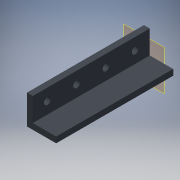
# Autodesk Inventor part: inside Angle beam
Saved by Autodesk Inventor 2016 (Build 200138000, 138)
## iProperties
Created: 2015-08-29
Part Number: inside Angle beam
Material: Generic
Description: ANGLE - 144 MM
Document SubType Name: Modeling
Designer: PTC
Density: 1 g/cm^3
Appearance: Default
Sending System: Creo  TM  2.0  (c) 2012
PROJECT: FTC
PTC_MATERIAL_NAME: METAL_ALUMINIUM_5052
NIKCONFIGCOUNT: 1
KIT: TETRIX
Author: phi
Autodesk Inventor part; units mm, degrees
ref_plane "FRONT" through (0, 0, 0) normal (0, 0, 1) x (1, 0, 0)
ref_plane "TOP" through (0, 0, 0) normal (0, 1, 0) x (-1, 0, 0)
ref_plane "RIGHT" through (0, 0, 0) normal (1, 0, 0) x (0, 1, 0)
ref_plane "Work Plane4" through (0, 0, 0) normal (0, 0, 1) x (1, 0, 0)
sketch "Sketch1" plane through (0, 0, 0) normal (0, 0, 1) x (1, 0, 0)
  line L0 (3.2, 16) -> (0, 16) projected
  line L1 (3.2, 3.2) -> (3.2, 14) projected
  line L2 (3.2, 14) -> (3.2, 16) projected
  line L3 (0, 16) -> (0, 14) projected
  line L4 (0, 14) -> (0, 0) projected
  line L5 (0, 0) -> (14, 0) projected
  line L6 (16, 0) -> (16, 3.2) projected
  line L7 (16, 3.2) -> (14, 3.2) projected
  line L8 (14, 3.2) -> (3.2, 3.2) projected
  line L9 (14, 0) -> (16, 0) projected
extrude "Extrusion1" add sketch "Sketch1" along normal blind 80
sketch "Sketch2" plane through (0, 0, 0) normal (-1, 0, 0) x (0, 0, 1)
  circle A0 centre (8, 9.6) radius 1.85 projected
  circle A1 centre (24, 9.6) radius 1.85 projected
  circle A2 centre (40, 9.6) radius 1.85 projected
  circle A3 centre (56, 9.6) radius 1.85 projected
  circle A4 centre (72, 9.6) radius 1.85 projected
  point P0 (0, 0)
hole "Hole1" at (0, 9.6, 8) at (0, 9.6, 24) at (0, 9.6, 40) at (0, 9.6, 56) at (0, 9.6, 72) direction (1, 0, 0) diameter 3.7 end through all
sketch "Sketch3" plane through (0, 0, 0) normal (0, -1, 0) x (1, 0, 0)
  circle A0 centre (9.6, 56) radius 1.85 projected
  circle A1 centre (9.6, 40) radius 1.85 projected
  circle A2 centre (9.6, 24) radius 1.85 projected
  circle A3 centre (9.6, 8) radius 1.85 projected
  circle A4 centre (9.6, 72) radius 1.85 projected
  point P0 (0, 0)
hole "Hole2" at (9.6, 0, 8) at (9.6, 0, 24) at (9.6, 0, 40) at (9.6, 0, 56) at (9.6, 0, 72) direction (0, 1, 0) diameter 3.7 end through all
fillet "Fillet1" radius 2 1 edges at (16, 1.6, 80)
fillet "Fillet2" radius 2 3 edges at (1.6, 16, 80) (1.6, 16, 0) (16, 1.6, 0)
body "Solid2"
